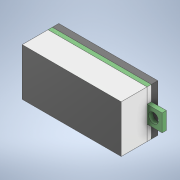
# Autodesk Inventor part: DC-Voltmeter-Red
Saved by Autodesk Inventor 2022.3 (Build 263350000, 350)
## iProperties
Part Number: DC-Voltmeter-Red
Material: Generic
Document SubType Name: Modeling
Designer: Masato Kubotera
Density: 1 g/cm^3
Appearance: Default
Catalog Web Link: https://akizukidenshi.com/catalog/g/gM-08468/
Author: Masato Kubotera
Autodesk Inventor part; units mm, degrees
ref_plane "YZ Plane" through (0, 0, 0) normal (1, 0, 0) x (0, 1, 0)
ref_plane "XZ Plane" through (0, 0, 0) normal (0, 1, 0) x (-1, 0, 0)
ref_plane "XY Plane" through (0, 0, 0) normal (0, 0, 1) x (1, 0, 0)
sketch "Sketch1" plane through (0, 0, 0) normal (0, 0, 1) x (1, 0, 0)
  line L0 (5.5, 11.5) -> (-5.5, 11.5)
  line L1 (-5.5, 11.5) -> (-5.5, -11.5)
  line L2 (-5.5, -11.5) -> (5.5, -11.5)
  line L3 (5.5, -11.5) -> (5.5, 11.5)
  line L4 (5.5, 11.5) -> (-5.5, -11.5) construction
  line L5 (-5.5, 11.5) -> (5.5, -11.5) construction
  line L6 (2, 11.5) -> (2, 15)
  line L7 (2, 15) -> (-2, 15)
  line L8 (-2, 15) -> (-2, 11.5)
  line L9 (5.5, 0) -> (-5.5, 0) construction
  line L10 (2, -11.5) -> (2, -15)
  line L11 (2, -15) -> (-2, -15)
  line L12 (-2, -15) -> (-2, -11.5)
  line L13 (0, 15) -> (0, -15) construction
  circle A0 centre (0, 13) radius 1.15
  circle A1 centre (0, -13) radius 1.15
  point P0 (0, 0)
  point P1 (0, 0)
  dimension "d0" = 23
  dimension "d1" = 11
  dimension "d2" = 2.3
  dimension "d3" = 4
  dimension "d4" = 3.5
  dimension "d5" = 26
  constraints: 28 end point, 8 midpoint, 5 symmetric about line, 3 perpendicular, 3 point on line, 2 centre point, 2 parallel, 1 horizontal, 1 vertical, 1 other
  measures "d0" distance of L2.end L0.start
  measures "d1" distance of L0.start L0.end
  measures "d2" diameter of A0
  measures "d3" distance of L11.start L12.start
  measures "d4" distance of L10.start L11.start
  measures "d5" distance of A1.centre A0.centre
extrude "Extrusion1" add sketch "Sketch1" along normal blind 1
extrude "Extrusion2" add sketch "Sketch1" along normal blind 7 separate body contours L3 L2 L1 L0
extrude "Extrusion3" add sketch "Sketch1" against normal blind 1.5 separate body contours L3 L2 L1 L0
body "Solid1"
body "Solid2"
body "Solid3"
